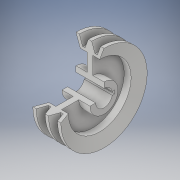
# Autodesk Inventor part: 410571040-3
Saved by Autodesk Inventor 2017 (Build 210142000, 142)
## iProperties
Part Number: 410571040-3
Material: 一般
Document SubType Name: Modeling
Designer: user
Density: 1 g/cm^3
Appearance: 預設
Author: user
Autodesk Inventor part; units mm, degrees
ref_plane "YZ Plane" through (0, 0, 0) normal (1, 0, 0) x (0, 1, 0)
ref_plane "XZ Plane" through (0, 0, 0) normal (0, 1, 0) x (-1, 0, 0)
ref_plane "XY Plane" through (0, 0, 0) normal (0, 0, 1) x (1, 0, 0)
sketch "草圖1" plane through (0, 0, 0) normal (0, 0, 1) x (1, 0, 0)
  line L0 (0, 0) -> (12.5, 0)
  line L1 (12.5, 0) -> (12.5, 12.5)
  line L2 (12.5, 12.5) -> (2.5, 12.5)
  line L3 (2.5, 12.5) -> (2.5, 28)
  line L4 (2.5, 28) -> (8.6783, 28)
  line L5 (8.6783, 28) -> (12.5, 38.5)
  line L6 (12.5, 38.5) -> (9.5, 38.5)
  line L7 (9.5, 38.5) -> (6.5882, 30.5)
  line L8 (6.5882, 30.5) -> (4.4118, 30.5)
  line L9 (4.4118, 30.5) -> (1.5, 38.5)
  line L10 (1.5, 38.5) -> (-0.2328, 38.5)
  line L11 (0, 0) -> (0, -1.5928)
  line L12 (0, 0) -> (-12.5, 0)
  line L13 (-12.5, 0) -> (-12.5, 12.5)
  line L14 (-12.5, 12.5) -> (-2.5, 12.5)
  line L15 (-2.5, 12.5) -> (-2.5, 28)
  line L16 (-2.5, 28) -> (-8.6783, 28)
  line L17 (-8.6783, 28) -> (-12.5, 38.5)
  line L18 (-12.5, 38.5) -> (-9.5, 38.5)
  line L19 (-9.5, 38.5) -> (-6.5882, 30.5)
  line L20 (-6.5882, 30.5) -> (-4.4118, 30.5)
  line L21 (-4.4118, 30.5) -> (-1.5, 38.5)
  line L22 (-1.5, 38.5) -> (-0.2328, 38.5)
  dimension "d10" = 25
  dimension "d11" = 3
  dimension "d12" = 8
  dimension "d13" = 5
  dimension "d14" = 25
  dimension "d15" = 40
  dimension "d16" = 8
  dimension "d17" = 38.5
  dimension "d18" = 28
  dimension "d19" = 12.5
  dimension "d20" = 40
  constraints: 46 end point, 10 symmetric about line, 4 perpendicular, 3 parallel, 2 horizontal, 1 collinear, 1 vertical
  measures "d10" distance of L5.end L17.end
  measures "d11" distance of L17.end L18.end
  measures "d12" distance of L6.end L9.end
  measures "d13" distance between parallel lines of L15 L3
  measures "d14" distance between parallel lines of L13 L1
  measures "d15" angle of L21 L19
  measures "d16" distance between parallel lines of L20 L22
  measures "d17" distance between parallel lines of L6 L0
  measures "d18" distance between parallel lines of L16 L12
  measures "d19" distance between parallel lines of L14 L12
  measures "d20" angle of L9 L21
revolve "迴轉1" add sketch "草圖1" angle 270 about axis through (0, 0, 0) along (-1, 0, 0)
sketch "草圖2" plane through (12.5, 0, 0) normal (1, 0, 0) x (0, 0, -1)
  arc A0 (7.3485, 1.5) -> (7.3485, -1.5) centre (0, 0) ccw
  line L0 (7.3485, -1.5) -> (9.5, -1.5)
  line L1 (9.5, -1.5) -> (9.5, 1.5)
  line L2 (9.5, 1.5) -> (7.3485, 1.5)
  dimension "d22" = 15
  dimension "d23" = 17
  dimension "d24" = 3
  dimension "d25" = 1.5
  constraints: 6 end point, 2 perpendicular, 2 point on circle, 1 centre point, 1 coincident, 1 horizontal
  measures "d22" diameter of A0
  measures "d24" distance of L0.end L1.end
  measures "d25" distance from line of point (0, 0) L0
extrude "擠出1" cut sketch "草圖2" against normal through all
